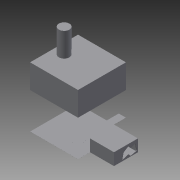
# Autodesk Inventor part: Harrison_Spill_Plumes
Saved by Autodesk Inventor 2013 SP2 (Build 170200200, 200)
## iProperties
Created: 2014-01-03
Part Number: Harrison_Spill_Plumes
Material: Generic
Document SubType Name: Modeling
Designer: mcgratta
Density: 1 g/cm^3
Author: mcgratta
Autodesk Inventor part; units mm, degrees
ref_plane "YZ Plane" through (0, 0, 0) normal (1, 0, 0) x (0, 1, 0)
ref_plane "XZ Plane" through (0, 0, 0) normal (0, 1, 0) x (-1, 0, 0)
ref_plane "XY Plane" through (0, 0, 0) normal (0, 0, 1) x (1, 0, 0)
sketch "Sketch1" plane through (0, 0, 0) normal (0, 0, 1) x (1, 0, 0)
  line L0 (0, 0) -> (2000, 0)
  line L1 (2000, 0) -> (2000, 2000)
  line L2 (2000, 2000) -> (0, 2000)
  line L3 (0, 2000) -> (0, 0)
  dimension "d0" = 2000
  dimension "d2" = 2000
  constraints: 8 end point, 2 parallel, 1 horizontal, 1 perpendicular
  measures "d0" distance of L1.end L2.end
  measures "d2" distance of L0.end L1.end
extrude "Extrusion1" add sketch "Sketch1" along normal blind 2500
shell "Shell1" thickness 1 removed faces 0
sketch "Sketch2" plane through (0, 0, 0) normal (0, -1, 0) x (1, 0, 0)
  line L0 (0, 0) -> (2000, 0) projected
  line L1 (2000, 0) -> (2000, 2500) projected
  line L2 (0, 0) -> (2000, 0)
  line L3 (2000, 0) -> (2000, 1500)
  line L4 (2000, 1500) -> (0, 1500)
  line L5 (0, 1500) -> (0, 0)
  dimension "d6" = 1500
  constraints: 8 end point, 2 parallel, 1 horizontal, 1 perpendicular, 1 point on line
  measures "d6" distance of L2.end L3.end
extrude "Extrusion2" cut sketch "Sketch2" along normal mid plane 2
sketch "Sketch3" plane through (2000, 0, 2500) normal (1, 0, 0) x (0, 0, -1)
  line L0 (2500, 2000) -> (0, 2000) projected
  line L1 (2500, 0) -> (1000, 0)
  line L2 (1000, 0) -> (1000, 2000)
  line L3 (1000, 2000) -> (2500, 2000)
  line L4 (2500, 2000) -> (2500, 0)
  dimension "d10" = 1500
  constraints: 8 end point, 2 parallel, 1 horizontal, 1 perpendicular, 1 point on line
  measures "d10" distance of L2.end L3.end
extrude "Extrusion3" cut sketch "Sketch3" along normal mid plane 2
sketch "Sketch4" plane through (0, 2000, 2500) normal (0, 1, 0) x (1, 0, 0)
  line L0 (0, 2500) -> (0, 0) projected
  line L1 (1999, 2500) -> (0, 2500)
  line L2 (0, 2500) -> (0, 1000)
  line L3 (0, 1000) -> (1999, 1000)
  line L4 (1999, 1000) -> (1999, 2500)
  dimension "d14" = 1500
  constraints: 8 end point, 2 parallel, 1 horizontal, 1 perpendicular, 1 point on line
  measures "d14" distance of L1.end L2.end
extrude "Extrusion4" cut sketch "Sketch4" against normal blind 2
sketch "Sketch5" plane through (0, 0, 2500) normal (-1, 0, 0) x (0, 0, 1)
  line L0 (-1000, 0) -> (0, 0) projected
  line L1 (-2500, 1998) -> (-1000, 1998)
  line L2 (-1000, 1998) -> (-1000, 0)
  line L3 (-1000, 0) -> (-2500, 0)
  line L4 (-2500, 0) -> (-2500, 1998)
  point P0 (-2500, 0)
  dimension "d18" = 1500
  constraints: 8 end point, 2 parallel, 1 horizontal, 1 perpendicular, 1 point on line
  measures "d18" distance of L2.end L3.end
extrude "Extrusion5" cut sketch "Sketch5" against normal blind 2
sketch "Sketch8" plane through (1999, 1, 1) normal (0, 0, 1) x (1, 0, 0)
  line L0 (-1997, 0) -> (0, 0) projected
  line L1 (0, 0) -> (0, 1997) projected
  line L2 (0, 500) -> (1000, 500)
  line L3 (1000, 500) -> (1000, 1500)
  line L4 (1000, 1500) -> (0, 1500)
  line L5 (0, 1500) -> (0, 500)
  point P0 (-1999, -1)
  dimension "d30" = 500
  dimension "d31" = 1000
  dimension "d65" = 1000
  constraints: 8 end point, 2 parallel, 1 horizontal, 1 perpendicular, 1 point on line
  measures "d30" distance between parallel lines of L0 L2
  measures "d31" distance of L2.end L3.end
  measures "d65" distance of L3.end L4.end
extrude "Extrusion8" add sketch "Sketch8" along normal blind 500
sketch "Sketch9" plane through (1999, 1, 501) normal (0, 0, 1) x (1, 0, 0)
  line L0 (-300, -1) -> (0, -1)
  line L1 (0, -1) -> (0, 1999)
  line L2 (0, 1999) -> (-300, 1999)
  line L3 (-300, 1999) -> (-300, -1)
  point P0 (-1999, -1)
  dimension "d34" = 2000
  dimension "d36" = 300
  constraints: 8 end point, 2 parallel, 1 horizontal, 1 perpendicular
  measures "d34" distance of L0.end L1.end
  measures "d36" distance of L0.start L0.end
extrude "Extrusion9" add sketch "Sketch9" against normal blind 1
sketch "Sketch10" plane through (0, 0, 2500) normal (0, 0, 1) x (1, 0, 0)
  line L0 (0, 0) -> (2000, 0) projected
  line L1 (0, 2000) -> (0, 0) projected
  circle A0 centre (420, 1000) radius 220
  dimension "d39" = 440
  dimension "d41" = 420
  dimension "d42" = 1000
  constraints: 1 centre point
  measures "d39" diameter of A0
  measures "d41" distance from line of A0.centre L1
  measures "d42" distance from line of L0 A0.centre
extrude "Extrusion10" add sketch "Sketch10" along normal blind 1000
sketch "Sketch12" plane through (1999, 501, 1) normal (-1, 0, 0) x (0, 0, 1)
  line L0 (0, 0) -> (0, 1000) projected
  line L1 (0, 0) -> (499, 0) projected
  line L2 (2, 998) -> (498, 998)
  line L3 (498, 998) -> (498, 2)
  line L4 (498, 2) -> (2, 2)
  line L5 (2, 2) -> (2, 998)
  point P0 (-1, -501)
  dimension "d51" = 496
  dimension "d53" = 2
  dimension "d54" = 996
  dimension "d55" = 2
  constraints: 8 end point, 2 parallel, 1 horizontal, 1 perpendicular
  measures "d51" distance between parallel lines of L5 L3
  measures "d53" distance between parallel lines of L5 L0
  measures "d54" distance between parallel lines of L4 L2
  measures "d55" distance between parallel lines of L1 L4
extrude "Extrusion12" cut sketch "Sketch12" against normal blind 980
sketch "Sketch15" plane through (1999, 503, 3) normal (0, 0, 1) x (1, 0, 0)
  line L0 (0, 996) -> (980, 996) projected
  line L1 (700, 371) -> (950, 371)
  line L2 (950, 371) -> (950, 621)
  line L3 (950, 621) -> (700, 621)
  line L4 (700, 621) -> (700, 371)
  line L5 (1000, -2) -> (1000, 998) projected
  point P0 (-1999, -503)
  dimension "d58" = 250
  dimension "d60" = 250
  dimension "d61" = 375
  dimension "d68" = 50
  constraints: 8 end point, 2 parallel, 1 horizontal, 1 perpendicular
  measures "d58" distance between parallel lines of L1 L3
  measures "d60" distance between parallel lines of L2 L4
  measures "d61" distance between parallel lines of L0 L3
  measures "d68" distance between parallel lines of L5 L2
extrude "Extrusion13" add sketch "Sketch15" along normal blind 15
sketch "Sketch17" plane through (2999, 501, 1) normal (1, 0, 0) x (0, 0, -1)
  line L0 (-290.0438, 399.6914) -> (-427.8429, 619.1492)
  line L1 (-427.8429, 619.1492) -> (-304.1531, 696.8149)
  line L2 (-304.1531, 696.8149) -> (-365.998, 887.0919)
  line L3 (-365.998, 887.0919) -> (-88.4488, 955.9914)
  line L4 (-88.4488, 955.9914) -> (-24.1101, 696.8149)
  line L5 (-24.1101, 696.8149) -> (-129.2782, 598.7345)
  line L6 (-129.2782, 598.7345) -> (-47.8269, 348.1347)
  line L7 (-47.8269, 348.1347) -> (-290.0438, 399.6914)
  point P0 (1, -501)
  constraints: 16 end point, 2 perpendicular, 1 parallel
extrude "Extrusion15" cut sketch "Sketch17" along normal mid plane 100
body "Solid1"
